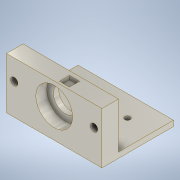
# Autodesk Inventor part: Soporte Extruder Izq
Saved by Autodesk Inventor 2021 (Build 250183000, 183)
## iProperties
Created: 2023-01-29
Part Number: Soporte Extruder Izq
Material: Titanio
Document SubType Name: Modeling
Designer: Diego.labarca
Density: 4.51 g/cm^3
Appearance: Titanio
Mass: 107.603 g
Surface Area: 114.42 cm^2
Volume: 23.8588 cm^3
Author: Diego.labarca
Autodesk Inventor part; units mm, degrees
ref_plane "YZ Plane" through (0, 0, 0) normal (1, 0, 0) x (0, 1, 0)
ref_plane "XZ Plane" through (0, 0, 0) normal (0, 1, 0) x (-1, 0, 0)
ref_plane "XY Plane" through (0, 0, 0) normal (0, 0, 1) x (1, 0, 0)
sketch "Boceto1" plane through (0, 0, 0) normal (0, 0, 1) x (1, 0, 0)
  line L0 (-26, 1.5) -> (26, 1.5)
  line L1 (26, 1.5) -> (26, -1.5)
  line L2 (26, -1.5) -> (-26, -1.5)
  line L3 (-26, -1.5) -> (-26, 1.5)
  line L4 (2.9301, 0) -> (0, 0)
  line L5 (0, 0) -> (0, 1.8389)
  dimension "d0" = 52
  dimension "d1" = 3
  constraints: 12 end point, 2 horizontal, 2 parallel, 2 perpendicular, 2 other
  measures "d0" distance of L1.end L2.end
  measures "d1" distance of L0.end L1.end
extrude "Extrusión1" add sketch "Boceto1" along normal blind 30
sketch "Boceto3" plane through (-26, 1.5, 0) normal (0, 1, 0) x (1, 0, 0)
  line L0 (52, 0) -> (52, -30) projected
  line L1 (0, -30) -> (52, -30) projected
  line L2 (52, 0) -> (47, 0)
  line L3 (47, 0) -> (47, -30)
  line L4 (47, -30) -> (52, -30)
  line L5 (52, -30) -> (52, 0)
  line L6 (0, 0) -> (0, -30) projected
  line L7 (0, 0) -> (5, 0)
  line L8 (5, 0) -> (5, -30)
  line L9 (5, -30) -> (0, -30)
  line L10 (0, -30) -> (0, 0)
  point P0 (26, 0)
  point P1 (5, -30)
  dimension "d4" = 5
  dimension "d5" = 5
  constraints: 16 end point, 4 parallel, 2 horizontal, 2 perpendicular, 2 point on line
  measures "d4" distance between parallel lines of L6 L8
  measures "d5" distance between parallel lines of L0 L3
extrude "Extrusión2" add sketch "Boceto3" along normal blind 25
sketch "Boceto5" plane through (0, 0, 30) normal (0, 0, 1) x (1, 0, 0)
  line L0 (-26, -1.5) -> (26, -1.5) projected
  line L1 (-26, -1.5) -> (-26, 26.5) projected
  line L2 (26, -1.5) -> (-26, -1.5)
  line L3 (-26, -1.5) -> (-26, 26.5)
  line L4 (-26, 26.5) -> (26, 26.5)
  line L5 (26, 26.5) -> (26, -1.5)
  point P0 (0, 0)
  constraints: 8 end point, 2 parallel, 1 horizontal, 1 perpendicular
extrude "Extrusión4" add sketch "Boceto5" along normal blind 3
sketch "Boceto6" plane through (0, 0, 33) normal (0, 0, 1) x (1, 0, 0)
  circle A0 centre (0, 14.5) radius 6.5
  line L0 (26, -1.5) -> (26, 26.5) projected
  line L1 (26, 26.5) -> (-26, 26.5) projected
  line L2 (-26, 26.5) -> (-26, -1.5) projected
  point P0 (0, 0)
  point P1 (2.0533, 26.5)
  point P2 (-6.2533, 26.5)
  dimension "d12" = 13
  dimension "d13" = 26
  dimension "d14" = 12
  dimension "d38" = 52
  constraints: 1 centre point
  measures "d12" diameter of A0
  measures "d13" distance from line of L0 A0.centre
  measures "d14" distance from line of A0.centre L1
  measures "d38" distance between parallel lines of L0 L2
extrude "Extrusión5" cut sketch "Boceto6" against normal up to surface (3 mm away)
sketch "Boceto7" plane through (-21, 1.5, 0) normal (0, 1, 0) x (1, 0, 0)
  circle A0 centre (33.5, -11.5916) radius 1.5
  circle A1 centre (8.5, -11.5916) radius 1.5
  line L0 (21, 0) -> (21, -4.282)
  dimension "d17" = 25
  dimension "d18" = 12.5
  dimension "d19" = 3
  dimension "d20" = 3
  constraints: 2 centre point, 2 end point, 1 vertical
  measures "d17" distance of A0.centre A1.centre
  measures "d18" distance from line of A0.centre L0
  measures "d19" diameter of A0
  measures "d20" diameter of A1
extrude "Extrusión6" cut sketch "Boceto7" against normal through all
sketch "Boceto9" plane through (0, 0, 33) normal (0, 0, 1) x (1, 0, 0)
  circle A0 centre (0, 14.5) radius 6.5 projected
  line L0 (-26, 26.5) -> (-26, -1.5) projected
  line L1 (26, 26.5) -> (-26, 26.5) projected
  line L2 (26, -1.5) -> (26, 26.5) projected
  line L3 (-26, -1.5) -> (26, -1.5) projected
  circle A1 centre (0, 14.5) radius 10
  point P0 (0, 0)
  point P1 (0, 26.5)
  dimension "d32" = 20
  constraints: 1 centre point, 1 coincident
  measures "d32" diameter of A1
extrude "Extrusión8" add sketch "Boceto9" along normal blind 6 contours L1 L2 L3 L0
sketch "Boceto8" plane through (0, 0, 39) normal (0, 0, 1) x (1, 0, 0)
  circle A0 centre (21.75, 15.395) radius 2
  circle A1 centre (-21.75, 15.395) radius 2
  line L0 (26, 26.5) -> (-26, 26.5) projected
  circle A2 centre (0, 14.5) radius 10 projected
  point P0 (0, 0)
  dimension "d23" = 4
  dimension "d24" = 4
  dimension "d25" = 43.5
  dimension "d35" = 11.105
  dimension "d36" = 11.105
  dimension "d37" = 21.75
  constraints: 2 centre point
  measures "d23" diameter of A0
  measures "d24" diameter of A1
  measures "d25" distance of A1.centre A0.centre
  measures "d35" distance from line of L0 A0.centre
  measures "d36" distance from line of L0 A1.centre
  measures "d37" horizontal distance of A0.centre A2.centre
extrude "Extrusión7" cut sketch "Boceto8" against normal blind 5 contours A0 | A1
sketch "Boceto10" plane through (-26, 26.5, 0) normal (0, 1, 0) x (1, 0, 0)
  circle A0 centre (30.3, -35) radius 2
  line L0 (52, 0) -> (52, -39) projected
  line L1 (52, -39) -> (0, -39) projected
  line L2 (27.55, -32.25) -> (33.05, -32.25)
  line L3 (33.05, -32.25) -> (33.05, -37.75)
  line L4 (33.05, -37.75) -> (27.55, -37.75)
  line L5 (27.55, -37.75) -> (27.55, -32.25)
  line L6 (27.55, -32.25) -> (33.05, -37.75) construction
  line L7 (33.05, -32.25) -> (27.55, -37.75) construction
  point P0 (26, 0)
  dimension "d39" = 21.7
  dimension "d41" = 4
  dimension "d45" = 5.5
  dimension "d46" = 5.5
  constraints: 12 end point, 2 midpoint, 2 parallel, 1 centre point, 1 coincident, 1 horizontal, 1 perpendicular
  measures "d39" distance from line of L0 A0.centre
  measures "d41" distance from line of L1 A0.centre
  measures "d45" distance of L3.end L4.end
  measures "d46" distance of L2.end L3.end
extrude "Extrusión9" cut sketch "Boceto10" against normal blind 2 contours A0 | L2 L3 L4 L5
sketch "Boceto11" plane through (26, -1.5, 0) normal (1, 0, 0) x (0, 0, -1)
  line L0 (-30, 28) -> (0, 28) projected
  line L1 (0, 28) -> (-30, 28)
  line L2 (-30, 28) -> (-30, 3)
  line L3 (-30, 3) -> (0, 3)
  line L4 (0, 3) -> (0, 28)
  point P0 (0, 1.5)
  dimension "d47" = 30
  dimension "d48" = 25
  constraints: 8 end point, 2 parallel, 1 horizontal, 1 perpendicular
  measures "d47" distance of L3.end L2.end
  measures "d48" distance of L2.end L1.end
extrude "Extrusión10" cut sketch "Boceto11" against normal up to surface (52 mm away)
sketch "Boceto12" plane through (-26, -1.5, 0) normal (0, -1, 0) x (1, 0, 0)
  circle A0 centre (26, 35.5) radius 2
  line L0 (0, 0) -> (0, 39) projected
  line L1 (52, 0) -> (52, 39) projected
  line L2 (0, 39) -> (52, 39) projected
  point P0 (26, 0)
  dimension "d51" = 4
  dimension "d52" = 52
  dimension "d53" = 26
  dimension "d54" = 3.5
  constraints: 1 centre point
  measures "d51" diameter of A0
  measures "d52" distance between parallel lines of L0 L1
  measures "d53" distance from line of L0 A0.centre
  measures "d54" distance from line of L2 A0.centre
extrude "Extrusión11" cut sketch "Boceto12" against normal blind 4
equation "\"d13\" = 0.5 * d38"
equation "\"d18\" = 0.5 * d17"
equation "\"d20\" = d19"
equation "\"d24\" = d23"
equation "\"d36\" = d35"
equation "\"d53\" = 0.5 * d52"
